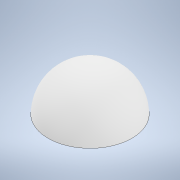
# Autodesk Inventor part: Globe Pommeau
Saved by Autodesk Inventor 2021 (Build 250183000, 183)
## iProperties
Created: 2020-09-20
Part Number: Globe Pommeau
Material: Générique
Document SubType Name: Modeling
Designer: Utilisateur
Density: 1 g/cm^3
Appearance: Par défaut
Author: Utilisateur
Autodesk Inventor part; units mm, degrees
ref_plane "YZ Plane" through (0, 0, 0) normal (1, 0, 0) x (0, 1, 0)
ref_plane "XZ Plane" through (0, 0, 0) normal (0, 1, 0) x (-1, 0, 0)
ref_plane "XY Plane" through (0, 0, 0) normal (0, 0, 1) x (1, 0, 0)
sketch "Esquisse1" plane through (0, 0, 0) normal (0, 0, 1) x (1, 0, 0)
  circle A0 centre (0, 0) radius 22.5
  line L0 (0, 26.2864) -> (0, -28.5844)
  line L1 (-28.231, 0) -> (38.5366, 0)
  circle A1 centre (0, 0) radius 22
  point P0 (22.5, 0)
  point P1 (0, 22.5)
  point P2 (-22, 0)
  point P3 (0, 22)
  point P4 (-22.5, 0)
  dimension "d0" = 45
  dimension "d2" = 44
  constraints: 4 end point, 2 centre point, 2 coincident, 1 horizontal, 1 vertical
  measures "d0" diameter of A0
  measures "d2" diameter of A1
revolve "Révolution1" add sketch "Esquisse1" angle 360 about axis through (0, 26.2864, 0) along (0, -1, 0) picked at (-21.9614, 3.3007) contours L0 A1 L1 A0
